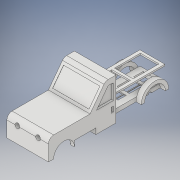
# Autodesk Inventor part: ambulance chassis
Saved by Autodesk Inventor 2019 (Build 230136000, 136)
## iProperties
Created: 2020-03-03
Part Number: ambulance chassis
Material: PC/ABS Plastic
Document SubType Name: Modeling
Designer: BT_3N8_25
Density: 0.357273 g/cm^3
Appearance: Smooth - White
Mass: 337.757 g
Surface Area: 1145 cm^2
Volume: 945.376 cm^3
Author: BT_3N8_25
Autodesk Inventor part; units mm, degrees
note: some values were not read from the file. Chosen so that the rebuilt part matches the saved one: direction of "Emboss1"; direction of "Emboss2"; direction of "Emboss4".
ref_plane "YZ Plane" through (0, 0, 0) normal (1, 0, 0) x (0, 1, 0)
ref_plane "XZ Plane" through (0, 0, 0) normal (0, 1, 0) x (-1, 0, 0)
sketch "Sketch1" plane through (0, 0, 0) normal (0, 0, 1) x (1, 0, 0)
  line L0 (-50.8, -25.4) -> (50.8, -25.4)
  line L1 (50.8, -25.4) -> (50.8, 25.4)
  line L2 (50.8, 25.4) -> (-50.8, 25.4)
  line L3 (-50.8, 25.4) -> (-50.8, -25.4)
  line L4 (-50.8, -25.4) -> (50.8, 25.4) construction
  line L5 (50.8, -25.4) -> (-50.8, 25.4) construction
  circle A0 centre (-25.4, 12.7) radius 5.715
  circle A1 centre (25.4, 12.7) radius 5.715
  point P0 (0, 0)
  dimension "d0" = 101.6
  dimension "d1" = 50.8
  dimension "d2" = 11.43
  dimension "d3" = 11.43
  dimension "d4" = 50.8
  dimension "d5" = 25.4
  dimension "d6" = 12.7
  constraints: 12 end point, 2 centre point, 2 midpoint, 2 parallel, 1 horizontal, 1 horizontal alignment, 1 perpendicular
  measures "d0" distance of L2.end L1.end
  measures "d1" distance of L0.end L1.end
  measures "d2" diameter of A0
  measures "d3" diameter of A1
  measures "d4" distance of A1.centre A0.centre
  measures "d5" distance from line of L1 A1.centre
  measures "d6" distance from line of L2 A0.centre
extrude "Extrusion1" add sketch "Sketch1" against normal blind 101.6
sketch "Sketch2" plane through (50.8, -25.4, 0) normal (1, 0, 0) x (0, 0, -1)
  line L0 (0, 0) -> (101.6, 0) projected
  arc A0 (63.5, 0) -> (12.7, 0) centre (38.1, 0) ccw
  line L1 (0, 0) -> (0, 50.8) projected
  point P0 (0, 25.4)
  dimension "d10" = 50.8
  dimension "d11" = 25.4
  dimension "d12" = 12.7
  constraints: 2 point on circle, 2 point on line, 1 centre point
  measures "d10" distance of A0.end A0.start
  measures "d11" radius of A0
  measures "d12" distance from line of L1 A0.end
extrude "Extrusion2" cut sketch "Sketch2" against normal through all
ref_plane "Work Plane2" through (0, 0, -139.7) normal (0, 0, -1) x (-1, 0, 0)
sketch "Sketch3" plane through (0, 0, -139.7) normal (0, 0, -1) x (-1, 0, 0)
  point P0 (0, 0)
sketch "Sketch4" plane through (0, 0, -139.7) normal (0, 0, -1) x (-1, 0, 0)
  line L0 (50.8, -25.4) -> (-50.8, -25.4)
  line L1 (-50.8, -25.4) -> (-50.8, 76.2)
  line L2 (-50.8, 76.2) -> (50.8, 76.2)
  line L3 (50.8, 76.2) -> (50.8, -25.4)
  circle A0 centre (-25.4, 12.7) radius 5.715 projected
  circle A1 centre (25.4, 12.7) radius 5.715 projected
  line L4 (-50.8, -25.4) -> (50.8, -25.4) projected
  line L5 (50.8, -25.4) -> (50.8, 25.4) projected
  line L6 (50.8, 25.4) -> (-50.8, 25.4) projected
  line L7 (-50.8, 25.4) -> (-50.8, -25.4) projected
  dimension "d16" = 101.6
  dimension "d19" = 101.6
  constraints: 8 end point, 2 collinear, 2 parallel, 1 horizontal, 1 perpendicular
  measures "d16" distance from line of L4.start L2
  measures "d19" distance of L1.end L2.end
sketch "Sketch5" plane through (0, 0, -101.6) normal (0, 0, -1) x (-1, 0, 0)
  circle A0 centre (-25.4, 12.7) radius 5.715 projected
  circle A1 centre (25.4, 12.7) radius 5.715 projected
  line L0 (-50.8, -25.4) -> (50.8, -25.4) projected
  line L1 (50.8, -25.4) -> (50.8, 25.4) projected
  line L2 (50.8, 25.4) -> (-50.8, 25.4) projected
  line L3 (-50.8, 25.4) -> (-50.8, -25.4) projected
  line L4 (-50.8, -25.4) -> (-50.8, 25.4) projected
  line L5 (-50.8, 25.4) -> (50.8, 25.4)
  line L6 (50.8, 25.4) -> (50.8, -25.4)
  line L7 (50.8, -25.4) -> (-50.8, -25.4)
  line L8 (-50.8, -25.4) -> (-50.8, 25.4)
  point P0 (-25.4, 0)
  constraints: 8 end point, 2 parallel, 1 horizontal, 1 perpendicular
loft "Loft1" add profiles "Sketch4" section 1 edges at (0, -25.4, -101.6) (-50.8, 0, -101.6) (0, 25.4, -101.6) (50.8, 0, -101.6) contours L0 L1 L6 L3 | L6 L1 L2 L3 | A0 | A1
sketch "Sketch6" plane through (50.8, -25.4, -139.7) normal (0, 0, -1) x (-1, 0, 0)
  line L0 (0, 0) -> (0, 101.6) projected
  line L1 (101.6, 50.8) -> (101.6, 0) projected
  line L2 (0, 101.6) -> (101.6, 101.6)
  line L3 (101.6, 101.6) -> (101.6, 0)
  line L4 (101.6, 0) -> (0, 0)
  line L5 (0, 0) -> (0, 101.6)
  point P0 (50.8, 25.4)
  constraints: 8 end point, 2 parallel, 1 horizontal, 1 perpendicular
extrude "Extrusion3" add sketch "Sketch6" along normal blind 25.4
sketch "Sketch7" plane through (50.8, -25.4, -165.1) normal (0, 0, -1) x (-1, 0, 0)
  line L0 (0, 0) -> (20.3858, 0)
  line L1 (101.6, 0) -> (81.28, 0)
  line L2 (50.8, 0) -> (50.8, 8.3294)
  line L3 (20.3858, 0) -> (35.6258, 0)
  line L4 (35.6258, 0) -> (35.6258, 10.16)
  line L5 (35.6258, 10.16) -> (20.3858, 10.16)
  line L6 (20.3858, 10.16) -> (20.3858, 0)
  line L7 (81.2142, 0) -> (65.9742, 0)
  line L8 (65.9742, 0) -> (65.9742, 10.16)
  line L9 (65.9742, 10.16) -> (81.2142, 10.16)
  line L10 (81.2142, 10.16) -> (81.2142, 0)
  point P0 (50.8, 25.4)
  constraints: 22 end point, 4 symmetric about line, 2 parallel, 1 collinear, 1 horizontal, 1 perpendicular, 1 vertical
fillet "Fillet1" radius 12.7 2 edges at (0, 76.2, -139.7) (0, 25.4, 0)
sketch "Sketch10" plane through (50.8, -25.4, -38.1) normal (1, 0, 0) x (0, 0, -1)
  arc A0 (-25.4, 50.8) -> (-38.1, 38.1) centre (-25.4, 38.1) ccw projected
  line L0 (-38.1, 0) -> (-38.1, 38.1) projected
  line L1 (-38.1, 0) -> (-25.4, 0) projected
  arc A1 (25.4, 0) -> (-25.4, 0) centre (0, 0) ccw projected
  line L2 (25.4, 0) -> (127, 0) projected
  line L3 (107.95, 101.6) -> (127, 101.6) projected
  arc A2 (107.95, 101.6) -> (97.79, 96.52) centre (107.95, 88.9) ccw projected
  line L4 (63.5, 50.8) -> (97.79, 96.52) projected
  line L5 (-25.4, 50.8) -> (63.5, 50.8) projected
  line L6 (79.4344, 50.8) -> (106.9976, 87.6275)
  line L7 (109.5395, 88.9) -> (117.475, 88.9)
  line L8 (120.65, 85.725) -> (120.65, 50.8)
  line L9 (120.65, 50.8) -> (79.4344, 50.8)
  arc A3 (109.5395, 88.9) -> (106.9976, 87.6275) centre (109.5395, 85.725) ccw
  arc A4 (120.65, 85.725) -> (117.475, 88.9) centre (117.475, 85.725) ccw
  line L10 (127, 101.6) -> (127, 0) projected
  point P0 (-38.1, 25.4)
  dimension "d37" = 0.057
  dimension "d38" = 15.9344
  dimension "d40" = 3.175
  constraints: 8 end point, 4 point on circle, 4 tangent, 2 centre point, 2 perpendicular, 2 point on line, 1 equal radius, 1 horizontal
  measures "d37" angle of L6 L4
  measures "d38" distance of L6.start L4.start
  measures "d40" radius of A3
emboss "Emboss1" sketch "Sketch10" operation cut depth 5.08 direction (-1, 0, 0) contours L6 A3 L7 A4 L8 L9
sketch "Sketch11" plane through (50.8, -25.4, -38.1) normal (1, 0, 0) x (0, 0, -1)
  line L0 (115.57, 39.0435) -> (120.65, 39.0435)
  line L1 (120.65, 39.0435) -> (120.65, 26.3435)
  line L2 (120.65, 26.3435) -> (115.57, 26.3435)
  line L3 (115.57, 26.3435) -> (115.57, 39.0435)
  line L4 (120.65, 50.8) -> (79.4344, 50.8) projected
  line L5 (120.65, 85.725) -> (120.65, 50.8) projected
  arc A0 (120.65, 85.725) -> (117.475, 88.9) centre (117.475, 85.725) ccw projected
  line L6 (109.5395, 88.9) -> (117.475, 88.9) projected
  arc A1 (109.5395, 88.9) -> (106.9976, 87.6275) centre (109.5395, 85.725) ccw projected
  line L7 (79.4344, 50.8) -> (106.9976, 87.6275) projected
  point P0 (-38.1, 25.4)
  dimension "d43" = 12.7
  dimension "d44" = 5.08
  constraints: 8 end point, 2 parallel, 1 collinear, 1 horizontal, 1 perpendicular
  measures "d43" distance of L0.end L1.end
  measures "d44" distance of L1.end L2.end
emboss "Emboss2" sketch "Sketch11" operation cut depth 5.08 direction (-1, 0, 0) contours L0 L1 L2 L3
sketch "Sketch13" plane through (-50.8, 25.4, -101.6) normal (0, 0.6, 0.8) x (1, 0, 0)
  line L0 (0, 57.15) -> (101.6, 57.15) projected
  line L1 (0, 0) -> (0, 57.15) projected
  line L2 (0, 0) -> (101.6, 0) projected
  line L3 (101.6, 0) -> (101.6, 57.15) projected
  line L4 (95.25, 50.8) -> (6.35, 50.8)
  line L5 (6.35, 50.8) -> (6.35, 6.35)
  line L6 (6.35, 6.35) -> (95.25, 6.35)
  line L7 (95.25, 6.35) -> (95.25, 50.8)
  point P0 (50.8, -81.28)
  dimension "d50" = 6.35
  constraints: 8 end point, 3 other
  measures "d50" distance between parallel lines of L0 L4
emboss "Emboss4" sketch "Sketch13" operation cut depth 0.508 direction (0, -0.6, -0.8) contours L7 L6 L5 L4
extrude "Extrusion7" add sketch "Sketch7" along normal blind 139.7
sketch "Sketch14" plane through (15.1742, -25.4, -165.1) normal (-1, 0, 0) x (0, 0, 1)
  line L0 (-40.64, 10.16) -> (-33.02, 10.16)
  line L1 (-68.58, 10.16) -> (-60.96, 10.16)
  line L2 (-109.22, 10.16) -> (-101.6, 10.16)
  line L3 (-139.7, 10.16) -> (-132.08, 10.16)
  line L4 (-132.08, 10.16) -> (-132.08, 0)
  line L5 (-132.08, 0) -> (-139.7, 0)
  line L6 (-139.7, 0) -> (-139.7, 10.16)
  line L7 (-109.22, 10.16) -> (-109.22, 7.62)
  line L8 (-109.22, 7.62) -> (-101.6, 7.62)
  line L9 (-101.6, 7.62) -> (-101.6, 10.16)
  line L10 (-68.58, 10.16) -> (-68.58, 7.62)
  line L11 (-68.58, 7.62) -> (-60.96, 7.62)
  line L12 (-60.96, 7.62) -> (-60.96, 10.16)
  line L13 (-40.64, 10.16) -> (-40.64, 7.62)
  line L14 (-40.64, 7.62) -> (-33.02, 7.62)
  line L15 (-33.02, 7.62) -> (-33.02, 10.16)
  point P0 (165.1, 25.4)
  point P1 (0, 0)
  dimension "d66" = 7.62
  dimension "d68" = 7.62
  dimension "d70" = 7.62
  dimension "d71" = 7.62
  dimension "d77" = 2.54
  constraints: 32 end point, 5 perpendicular, 4 parallel, 4 point on line, 1 horizontal, 1 vertical
  measures "d66" distance of L0.start L0.end
  measures "d68" distance of L1.start L1.end
  measures "d70" distance of L2.start L2.end
  measures "d71" distance of L4.end L5.end
  measures "d77" distance of L2.start L7.end
extrude "Extrusion8" add sketch "Sketch14" along normal up to next
fillet "Fillet2" radius 3.175 2 edges at (30.4142, -20.32, -304.8) (-30.4142, -20.32, -304.8)
sketch "Sketch15" plane through (50.8, -25.4, -165.1) normal (0, 0, -1) x (-1, 0, 0)
  line L0 (20.3858, 10.16) -> (35.6258, 10.16) projected
  line L1 (65.9742, 10.16) -> (81.2142, 10.16) projected
  line L2 (35.6258, 10.16) -> (65.9742, 10.16)
  line L3 (41.0292, 10.16) -> (42.9768, 10.16)
  line L4 (42.9768, 10.16) -> (42.9768, 9.0842)
  line L5 (42.9768, 9.0842) -> (41.0292, 9.0842)
  line L6 (41.0292, 9.0842) -> (41.0292, 10.16)
  line L7 (57.3707, 10.16) -> (59.1115, 10.16)
  line L8 (59.1115, 10.16) -> (59.1115, 9.0842)
  line L9 (59.1115, 9.0842) -> (57.3707, 9.0842)
  line L10 (57.3707, 9.0842) -> (57.3707, 10.16)
  point P0 (50.8, 25.4)
  constraints: 18 end point, 4 parallel, 3 horizontal, 3 point on line, 2 perpendicular
extrude "Extrusion9" add sketch "Sketch15" along normal blind 139.7
sketch "Sketch18" plane through (50.8, -25.4, -165.1) normal (0, 0, -1) x (-1, 0, 0)
  point P0 (50.8, 25.4)
sketch "Sketch24" plane through (30.4142, -25.4, -165.1) normal (1, 0, 0) x (0, 0, -1)
  line L0 (77.5614, 0.0121) -> (128.3614, 0)
  arc A0 (128.3614, 0) -> (77.5614, 0.0121) centre (102.9614, 0.006) ccw
  line L1 (136.525, 0) -> (136.525, 10.16) projected
  line L2 (77.5614, 0.0121) -> (69.408, 0.0121)
  line L3 (128.3614, 0) -> (136.525, 0)
  arc A1 (136.525, 0) -> (69.408, 0.0121) centre (102.9665, 0) ccw
  point P0 (-165.1, 25.4)
  dimension "d99" = 50.8
  dimension "d100" = 25.4
  dimension "d101" = 8.1534
  constraints: 6 end point, 4 point on circle, 2 centre point, 1 tangent
  measures "d99" distance of L0.start L0.end
  measures "d100" radius of A0
  measures "d101" distance of L0.start L2.end
extrude "Extrusion18" add sketch "Sketch24" along normal blind 12.7 contours L2 A1 L3 A0
sketch "Sketch25" plane through (-30.4142, -25.4, -165.1) normal (-1, 0, 0) x (0, 0, 1)
  arc A0 (-77.5614, 0.0121) -> (-128.3614, 0) centre (-102.9614, 0.006) ccw
  arc A1 (-69.408, 0.0121) -> (-70.983, 10.16) centre (-102.9665, 0) ccw projected
  arc A2 (-69.408, 0.0121) -> (-136.525, 0) centre (-102.9665, 0.006) ccw
  line L0 (-136.525, 0) -> (-128.3614, 0)
  line L1 (-77.5614, 0.0121) -> (-69.408, 0.0121)
  line L2 (0, 0) -> (-128.3614, 0) projected
  point P0 (165.1, 25.4)
  dimension "d104" = 50.8
  constraints: 4 end point, 4 point on circle, 2 centre point, 2 horizontal, 1 other
  measures "d104" distance of L0.end L1.start
extrude "Extrusion19" add sketch "Sketch25" along normal blind 12.7
sketch "Sketch26" plane through (50.8, -25.4, -165.1) normal (0, 0, -1) x (-1, 0, 0)
  line L0 (65.9742, 10.16) -> (81.2142, 10.16) projected
  line L1 (20.3858, 40.64) -> (81.2142, 40.64)
  line L2 (20.3858, 40.64) -> (81.2142, 40.64)
  line L3 (81.2142, 40.64) -> (81.2142, 44.45)
  line L4 (81.2142, 44.45) -> (20.3858, 44.45)
  line L5 (20.3858, 44.45) -> (20.3858, 40.64)
  line L6 (20.3858, 44.45) -> (28.0058, 44.45)
  line L7 (28.0058, 44.45) -> (28.0058, 40.64)
  line L8 (81.2142, 44.45) -> (73.5942, 44.45)
  line L9 (73.5942, 44.45) -> (73.5942, 40.64)
  line L10 (50.8, 44.45) -> (48.26, 44.45)
  line L11 (50.8, 44.45) -> (53.34, 44.45)
  line L12 (53.34, 44.45) -> (53.34, 40.64)
  line L13 (48.26, 44.45) -> (48.26, 40.64)
  point P0 (50.8, 25.4)
  point P1 (20.3858, 10.16)
  dimension "d110" = 3.81
  constraints: 26 end point, 8 point on line, 5 perpendicular, 2 horizontal, 2 parallel, 1 midpoint
  measures "d110" distance of L3.end L2.end
extrude "Extrusion23" add sketch "Sketch26" along normal blind 139.7 contours L5 L4 L7 L1 | L9 L4 L3 L1
sketch "Sketch30" plane through (22.7942, 15.24, -165.1) normal (-1, 0, 0) x (0, 0, 1)
  line L0 (-139.7, 0) -> (-139.7, 3.81) projected
  line L1 (0, 0) -> (-139.7, 0) projected
  line L2 (-139.7, 3.81) -> (-133.35, 3.81)
  line L3 (-133.35, 3.81) -> (-133.35, 0)
  line L4 (-133.35, 0) -> (-139.7, 0)
  line L5 (-139.7, 0) -> (-139.7, 3.81)
  line L6 (-69.85, 3.81) -> (-63.5, 3.81)
  line L7 (-63.5, 3.81) -> (-63.5, 0)
  line L8 (-63.5, 0) -> (-69.85, 0)
  line L9 (-69.85, 0) -> (-69.85, 3.81)
  point P0 (165.1, -15.24)
  dimension "d124" = 6.35
  dimension "d127" = 6.35
  constraints: 16 end point, 4 parallel, 2 horizontal, 2 perpendicular, 2 point on line
  measures "d124" distance of L3.end L4.end
  measures "d127" distance of L7.end L8.end
extrude "Extrusion24" add sketch "Sketch30" along normal up to next
sketch "Sketch32" plane through (-50.8, -25.4, -38.1) normal (-1, 0, 0) x (0, 0, 1)
  line L0 (-25.4, 0) -> (-127, 0) projected
  line L1 (-25.4, 0) -> (-30.48, 0)
  line L2 (-25.4, 0) -> (-49.2813, 0)
  line L3 (-25.4, 0) -> (-52.4867, 0)
  line L4 (-52.4867, 0) -> (-52.4867, 14.1965)
  line L5 (-52.4867, 14.1965) -> (-25.4, 14.1965)
  line L6 (-25.4, 14.1965) -> (-25.4, 0)
  point P0 (38.1, 25.4)
  constraints: 12 end point, 2 horizontal, 2 parallel, 1 perpendicular, 1 point on line
extrude "Extrusion25" cut sketch "Sketch32" against normal through all
sketch "Sketch34" plane through (-50.8, -25.4, -63.5) normal (0, 0, -1) x (-1, 0, 0)
  line L0 (-101.6, 0) -> (0, 0) projected
  line L1 (0, 14.1965) -> (-101.6, 14.1965) projected
  line L2 (-92.6008, 0) -> (-11.517, 0)
  line L3 (-11.517, 0) -> (-11.517, 14.1965)
  line L4 (-11.517, 14.1965) -> (-92.6008, 14.1965)
  line L5 (-92.6008, 14.1965) -> (-92.6008, 0)
  point P0 (-50.8, 25.4)
  constraints: 8 end point, 2 parallel, 2 point on line, 1 horizontal, 1 perpendicular
extrude "Extrusion26" cut sketch "Sketch34" against normal blind 2.54
sketch "Sketch35" plane through (-50.8, -25.4, -60.96) normal (0, 0, -1) x (-1, 0, 0)
  line L0 (-92.6008, 14.1965) -> (-11.517, 14.1965) projected
  line L1 (-11.517, 11.0716) -> (-92.6008, 11.0716) projected
  line L2 (-92.6008, 14.1965) -> (-11.517, 14.1965)
  line L3 (-11.517, 14.1965) -> (-11.517, 11.0716)
  line L4 (-11.517, 11.0716) -> (-92.6008, 11.0716)
  line L5 (-92.6008, 11.0716) -> (-92.6008, 14.1965)
  point P0 (-50.8, 25.4)
  constraints: 8 end point, 2 parallel, 1 horizontal, 1 perpendicular
extrude "Extrusion27" cut sketch "Sketch35" against normal blind 2.54
sketch "Sketch36" plane through (30.4142, -25.4, -165.1) normal (1, 0, 0) x (0, 0, -1)
  arc A0 (79.6793, 10.16) -> (77.5614, 0.0121) centre (102.9614, 0.006) ccw projected
  line L0 (77.5614, 0.0121) -> (102.9614, 0)
  line L1 (0, 0) -> (128.3614, 0) projected
  circle A1 centre (102.9614, 0) radius 3.81
  point P0 (-165.1, 25.4)
  dimension "d137" = 25.4
  dimension "d138" = 7.62
  constraints: 2 end point, 1 centre point, 1 coincident, 1 point on line
  measures "d137" distance of L0.start L0.end
  measures "d138" diameter of A1
extrude "Extrusion28" cut sketch "Sketch36" against normal through all
sketch "Sketch37" plane through (-50.8, -25.4, -90.5867) normal (0, 0, 1) x (1, 0, 0)
  line L0 (0, 0) -> (0, 14.1965) projected
  line L1 (101.6, 0) -> (0, 0) projected
  line L2 (0, 14.1965) -> (101.6, 14.1965)
  line L3 (101.6, 14.1965) -> (101.6, 0)
  line L4 (101.6, 0) -> (0, 0)
  line L5 (0, 0) -> (0, 14.1965)
  point P0 (50.8, 25.4)
  constraints: 8 end point, 2 parallel, 1 horizontal, 1 perpendicular
extrude "Extrusion29" cut sketch "Sketch37" against normal blind 25.4
equation "\"d3\" = d2"
body "Solid1"
